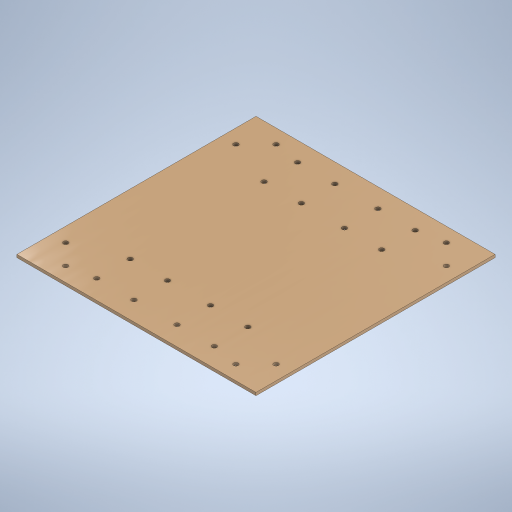
# Autodesk Inventor part: L1 Wood Base Iteration 1
Saved by Autodesk Inventor 2024 (Build 280153000, 153)
## iProperties
Created: 2023-06-26
Part Number: L1 Wood Base Iteration 1
Material: Aluminum 6061
Document SubType Name: Modeling
Designer: AdminForWorker
Density: 2.7 g/cm^3
Appearance: Brindle
Title: base
Author: AdminForWorker
Autodesk Inventor part; units mm, degrees
ref_plane "YZ Plane" through (0, 0, 0) normal (1, 0, 0) x (0, 1, 0)
ref_plane "XZ Plane" through (0, 0, 0) normal (0, 1, 0) x (-1, 0, 0)
ref_plane "XY Plane" through (0, 0, 0) normal (0, 0, 1) x (1, 0, 0)
sketch "Sketch3" plane through (0, 0, 0) normal (0, 1, 0) x (-1, 0, 0)
  line L0 (125, -125) -> (-125, -125)
  line L1 (-125, -125) -> (-125, 125)
  line L2 (-125, 125) -> (125, 125)
  line L3 (125, 125) -> (125, -125)
  line L4 (125, -125) -> (-125, 125) construction
  line L5 (-125, -125) -> (125, 125) construction
  point P0 (0, 0)
  dimension "L0" = 250
  dimension "W0" = 250
  constraints: 12 end point, 2 midpoint, 2 parallel, 1 horizontal, 1 perpendicular
  measures "L0" distance of L1.end L2.end
  measures "W0" distance of L0.end L1.end
extrude "Main Body Extrusion" add sketch "Sketch3" along normal blind 3
sketch "Sketch11" plane through (0, 3, 0) normal (0, 1, 0) x (1, 0, 0)
  circle A0 centre (61.4917, -70.0531) radius 2.5
  circle A1 centre (22.4917, -105.0531) radius 2.5
  circle A2 centre (-22.5083, -70.0531) radius 2.5
  circle A3 centre (-61.5083, -105.0531) radius 2.5
  circle A4 centre (-22.5083, -105.0531) radius 2.5
  circle A5 centre (61.4917, -105.0531) radius 2.5
  circle A6 centre (-61.5083, -70.0531) radius 2.5
  circle A7 centre (61.4917, 104.9469) radius 2.5
  circle A8 centre (61.4917, 69.9469) radius 2.5
  circle A9 centre (22.4917, 104.9469) radius 2.5
  circle A10 centre (-22.5083, 69.9469) radius 2.5
  circle A11 centre (-61.5083, 104.9469) radius 2.5
  circle A12 centre (-22.5083, 104.9469) radius 2.5
  circle A13 centre (22.4917, -70.0531) radius 2.5
  circle A14 centre (22.4917, 69.9469) radius 2.5
  line L0 (-125.0083, 124.9469) -> (124.9917, 124.9469)
  line L1 (124.9917, 124.9469) -> (124.9917, -125.0531)
  line L2 (124.9917, -125.0531) -> (-125.0083, -125.0531)
  line L3 (-125.0083, -125.0531) -> (-125.0083, 124.9469)
  point P0 (0, 0)
  point P1 (-61.5083, 69.9469)
  dimension "d86" = 250
  dimension "d87" = 250
  constraints: 15 centre point, 15 coincident, 8 end point, 2 parallel, 1 horizontal, 1 horizontal alignment, 1 perpendicular, 1 vertical alignment
  measures "d86" distance of L1.end L2.end
  measures "d87" distance of L0.end L1.end
hole "Bracket Holes" at (61.4917, 3, 70.0531) at (22.4917, 3, 105.0531) at (-22.5083, 3, 70.0531) at (-61.5083, 3, 105.0531) at (-22.5083, 3, 105.0531) at (61.4917, 3, 105.0531) at (-61.5083, 3, 70.0531) at (61.4917, 3, -104.9469) at (61.4917, 3, -69.9469) at (22.4917, 3, -104.9469) at (-22.5083, 3, -69.9469) at (-61.5083, 3, -104.9469) at (-22.5083, 3, -104.9469) at (22.4917, 3, 70.0531) at (22.4917, 3, -69.9469) at (-61.5083, 3, -69.9469) direction (0, -1, 0) diameter 5 end through all
sketch "Sketch12" plane through (0, 3, 0) normal (0, 1, 0) x (1, 0, 0)
  line L0 (85, -115) -> (115, -115)
  line L1 (115, -115) -> (115, -110.5263)
  line L2 (105, -105) -> (85, -105)
  line L3 (85, -105) -> (85, -115)
  line L4 (115, -85) -> (105, -85)
  line L5 (105, -85) -> (105, -105)
  line L6 (110.5263, -115) -> (115, -115)
  line L7 (115, -115) -> (115, -85)
  line L8 (125, -125) -> (125, 125) projected
  line L9 (-125, -125) -> (125, -125) projected
  line L10 (115, 115) -> (110.5263, 115)
  line L11 (115, 110.5263) -> (115, 115)
  line L12 (105, 105) -> (105, 85)
  line L13 (105, 85) -> (115, 85)
  line L14 (115, 85) -> (115, 115)
  line L15 (85, 115) -> (85, 105)
  line L16 (85, 105) -> (105, 105)
  line L17 (115, 115) -> (85, 115)
  line L18 (-115, 115) -> (-115, 110.5263)
  line L19 (-110.5263, 115) -> (-115, 115)
  line L20 (-105, 105) -> (-85, 105)
  line L21 (-85, 105) -> (-85, 115)
  line L22 (-85, 115) -> (-115, 115)
  line L23 (-115, 85) -> (-105, 85)
  line L24 (-105, 85) -> (-105, 105)
  line L25 (-115, 115) -> (-115, 85)
  line L26 (-115, -115) -> (-110.5263, -115)
  line L27 (-115, -110.5263) -> (-115, -115)
  line L28 (-105, -105) -> (-105, -85)
  line L29 (-105, -85) -> (-115, -85)
  line L30 (-115, -85) -> (-115, -115)
  line L31 (-85, -115) -> (-85, -105)
  line L32 (-85, -105) -> (-105, -105)
  line L33 (-115, -115) -> (-85, -115)
  point P0 (0, 0)
  point P1 (89, -110)
  point P2 (110, -89)
  point P3 (110, -85)
  point P4 (85, 110)
  point P5 (89, 110)
  point P6 (110, 89)
  point P7 (-110, 85)
  point P8 (-110, 89)
  point P9 (-89, 110)
  point P10 (-85, -110)
  point P11 (-89, -110)
  point P12 (-110, -89)
  dimension "d95" = 30
  dimension "d96" = 30
  dimension "d97" = 20
  dimension "d98" = 20
  dimension "d99" = 10
  dimension "d100" = 10
  dimension "d101" = 4
  dimension "d102" = 5
  dimension "d103" = 5
  dimension "d104" = 4
  dimension "d107" = 360
  constraints: 64 end point, 8 point on line, 4 parallel, 2 horizontal, 2 perpendicular, 1 midpoint, 81 other
  measures "d95" distance of L0.start L0.end
  measures "d96" distance of L6.end L4.start
  measures "d97" distance of L2.start L2.end
  measures "d98" distance of L4.end L2.start
  measures "d99" distance between parallel lines of L8 L7
  measures "d100" distance between parallel lines of L9 L0
  measures "d101" distance from line of L3 point (89, -110)
  measures "d102" distance from line of L0 point (89, -110)
  measures "d103" distance from line of L5 point (110, -89)
  measures "d104" distance of point (110, -85) point (110, -89)
hole "Hole4" at (89, 3, 110) at (110, 3, 89) at (89, 3, -110) at (110, 3, -89) at (-110, 3, -89) at (-89, 3, -110) at (-89, 3, 110) at (-110, 3, 89) direction (0, -1, 0) diameter 5 end through all
